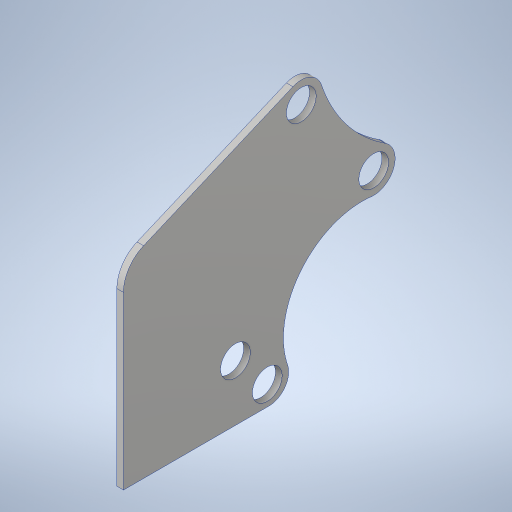
# Autodesk Inventor part: GI - 001
Saved by Autodesk Inventor 2023.4 (Build 274418000, 418)
## iProperties
Created: 2025-01-17
Part Number: GI - 001
Material: Aluminum 6061
Document SubType Name: Modeling
Designer: mavericks
Density: 2.7 g/cm^3
Appearance: Aluminum - Flat
Author: mavericks
Autodesk Inventor part; units mm, degrees
ref_plane "YZ Plane" through (0, 0, 0) normal (1, 0, 0) x (0, 1, 0)
ref_plane "XZ Plane" through (0, 0, 0) normal (0, 1, 0) x (-1, 0, 0)
ref_plane "XY Plane" through (0, 0, 0) normal (0, 0, 1) x (1, 0, 0)
sketch "Sketch2" plane through (0, 0, 0) normal (1, 0, 0) x (0, 1, 0)
  line L0 (63.5, 38.1) -> (-63.5, 38.1) construction
  line L1 (-63.5, 38.1) -> (-63.5, -38.1) construction
  line L2 (-63.5, -38.1) -> (63.5, -38.1) construction
  line L3 (63.5, -38.1) -> (63.5, 38.1) construction
  line L4 (63.5, 38.1) -> (-63.5, -38.1) construction
  line L5 (-63.5, 38.1) -> (63.5, -38.1) construction
  line L6 (-63.5, 38.1) -> (-76.2, 38.1) construction
  line L7 (-76.2, 38.1) -> (-76.2, -266.7) construction
  line L8 (-76.2, -266.7) -> (-63.5, -266.7) construction
  line L9 (-63.5, -266.7) -> (-63.5, 38.1) construction
  circle A0 centre (22.0517, -365.3177) radius 57.15 construction
  circle A1 centre (-50.8, -100.5497) radius 15.875 construction
  circle A2 centre (-15.875, -69.85) radius 25.4 construction
  circle A3 centre (76.2, -203.2) radius 63.5 construction
  circle A4 centre (76.2, -203.2) radius 14.2875
  circle A5 centre (166.2946, -133.35) radius 38.1 construction
  circle A6 centre (166.2946, -133.35) radius 14.2875
  circle A7 centre (-50.8, -100.5497) radius 14.2875
  circle A8 centre (-15.875, -69.85) radius 14.2875
  line L10 (-69.85, 38.1) -> (-69.85, -102.1372)
  arc A9 (-50.8, -121.1872) -> (-44.2424, -120.1177) centre (-50.8, -100.5497) ccw
  arc A10 (55.692, -200.8917) -> (93.5118, -214.4342) centre (76.2, -203.2) ccw
  arc A11 (172.8612, -152.9149) -> (185.307, -125.3228) centre (166.2946, -133.35) ccw
  arc A12 (55.692, -200.8917) -> (-44.2424, -120.1177) centre (-20.0298, -192.3686) ccw
  line L11 (-69.85, 38.1) -> (95.25, 38.1)
  line L12 (124.4998, 18.6995) -> (185.307, -125.3228)
  arc A13 (172.8612, -152.9149) -> (93.5118, -214.4342) centre (221.353, -297.3944) ccw
  arc A14 (124.4998, 18.6995) -> (95.25, 38.1) centre (95.25, 6.35) ccw
  arc A15 (-69.85, -102.1372) -> (-50.8, -121.1872) centre (-50.8, -102.1372) ccw
  point P0 (0, 0)
  dimension "d2" = 127
  dimension "d3" = 76.2
  dimension "d4" = 12.7
  dimension "d5" = 304.8
  dimension "d6" = 114.3
  dimension "d7" = 31.75
  dimension "d8" = 50.8
  dimension "d9" = 127
  dimension "d10" = 152.4
  dimension "d11" = 28.575
  dimension "d12" = 31.75
  dimension "d13" = 25.4
  dimension "d14" = 46.4998
  dimension "d15" = 47.625
  dimension "d16" = 165.1
  dimension "d17" = 76.2
  dimension "d18" = 114.0003
  dimension "d19" = 69.85
  dimension "d20" = 28.575
  dimension "d21" = 28.575
  dimension "d22" = 28.575
  dimension "d23" = 6.35
  dimension "d24" = 6.35
  dimension "d25" = 6.35
  dimension "d26" = 76.2
  dimension "d28" = 165.1
  dimension "d29" = 152.4
  dimension "d30" = 31.75
  dimension "d35" = 19.05
  constraints: 26 end point, 16 centre point, 14 point on circle, 10 tangent, 4 coincident, 4 parallel, 3 midpoint, 3 perpendicular, 2 horizontal
  measures "d2" distance of L2.end L1.end
  measures "d3" distance of L1.end L0.end
  measures "d4" distance of L8.end L7.end
  measures "d5" distance of L7.end L6.end
  measures "d6" diameter of A0
  measures "d7" diameter of A1
  measures "d8" diameter of A2
  measures "d9" diameter of A3
  measures "d10" distance from line of A3.centre L7
  measures "d11" diameter of A4
  measures "d12" distance from line of A2.centre L2
  measures "d13" distance from line of L7 A1.centre
  measures "d14" distance of A2.centre A1.centre
  measures "d15" distance from line of L9 A2.centre
  measures "d16" distance from line of L2 A3.centre
  measures "d17" diameter of A5
  measures "d18" distance of A3.centre A5.centre
  measures "d19" vertical distance of A5.centre A3.centre
  measures "d20" diameter of A6
  measures "d21" diameter of A7
  measures "d22" diameter of A8
  measures "d23" radial gap between concentric circles of A7 A9
  measures "d24" radial gap between concentric circles of A4 A10
  measures "d25" radial gap between concentric circles of A6 A11
  measures "d26" radius of A12
  measures "d28" distance of L11.end L10.start
  measures "d29" radius of A13
  measures "d30" radius of A14
  measures "d35" radius of A15
extrude "Extrusion1" add sketch "Sketch2" along normal blind 6.35
body "Solid1"
